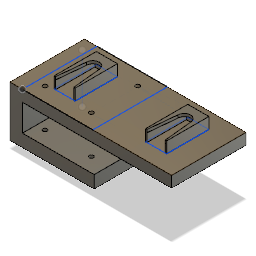
socle stepper 1 (Autodesk Fusion 360 design; units mm, degrees)
Autodesk Fusion 360 part; units mm, degrees
note: some values were not read from the file. Chosen so that the rebuilt part matches the saved one: which face or edge a step refers to. Set by a fixed rule: which sketch regions a step uses.
sketch "Sketch2" plane through (0, 0, 0) normal (0, 1, 0) x (1, 0, 0) in component "junction"
  line L0 (0, 0) -> (100, 0)
  line L1 (100, 0) -> (100, 50)
  line L2 (100, 50) -> (0, 50)
  line L3 (0, 50) -> (0, 0)
  line L4 (100, 50) -> (78.0729, 50)
sketch "Sketch3" plane through (0, 0, 0) normal (1, 0, 0) x (0, 0, -1) in component "junction"
  line L0 (0, 29.5553) -> (50.0119, 29.5553)
  line L1 (50.0119, 29.5553) -> (50.0119, 0)
  line L2 (50.0119, 0) -> (0, 0)
  line L3 (0, 0) -> (0, 29.5553)
sketch "Sketch4" plane through (0, 2.5, -25.0059) normal (1, 0, 0) x (0, 0, -1) in component "junction"
sketch "Sketch5" plane through (0, 0, 0) normal (1, 0, 0) x (0, 1, 0) in component "junction"
  line L0 (30, -50) -> (-5, -50)
extrude "Extrude1" add sketch "Sketch2" along normal blind 10 in component "junction"
extrude "Extrude2" add sketch "Sketch3" along normal blind 5 in component "junction"
extrude "Extrude3" cut 1 faces at (36.6667, 10, -33.3333) along direction (0, -1, 0) blind 5 in component "junction"
extrude "Extrude4" add 1 faces at (36.6667, 5, -33.3333) along direction (0, 1, 0) blind 4 in component "junction"
extrude "Extrude5" add 1 faces at (1.6667, 29.5553, -16.6706) along direction (0, 1, 0) blind 20 in component "junction"
extrude "Extrude6" add 1 faces at (5, 36.0369, -33.3373) along direction (1, 0, 0) blind 4 in component "junction"
extrude "Extrude7" cut 1 faces at (6, 49.5553, -33.3413) along direction (0, -1, 0) blind 10 in component "junction"
extrude "Extrude8" add 1 faces at (6, 39.5553, -33.3413) along direction (0, 1, 0) blind 0.055 in component "junction"
extrude "Extrude9" add 1 faces at (6, 39.6103, -33.3413) along direction (0, 1, 0) blind 0.39 in component "junction"
sketch "Sketch6" plane through (0, 40.0003, 0) normal (0, 1, 0) x (-1, 0, 0) in component "junction"
  line L0 (0, -50.0119) -> (0, 0)
  line L1 (0, 0) -> (-9, 0)
  line L2 (-9, 0) -> (-9, -50.0119)
  line L3 (-9, -50.0119) -> (0, -50.0119)
  line L4 (-9, -50.0119) -> (-115, -50.0119)
  line L5 (-115, -50.0119) -> (-115, 0)
  line L6 (-115, 0) -> (-9, 0)
  line L7 (-9, 0) -> (-9, -50.0119)
  line L8 (-9, 0) -> (-100, 0)
extrude "Extrude10" cut 1 faces at (100, 3, -16.6667) along direction (-1, 0, 0) blind 40 in component "junction"
extrude "Extrude11" add sketch "Sketch6" along normal blind 8 in component "junction"
extrude "Extrude12" add 1 faces at (44.3333, 40.0003, -33.3413) along direction (0, -1, 0) blind 12 in component "junction"
extrude "Extrude13" cut 1 faces at (76.6667, 48.0003, -33.3413) along direction (0, -1, 0) blind 12 in component "junction"
sketch "Sketch7" plane through (0, 0, 0) normal (0, -1, 0) x (1, 0, 0) in component "junction"
  line L0 (60, -50) -> (60, 0)
  line L1 (60, 0) -> (0, 0)
  line L2 (0, 0) -> (0, -50.0119)
  line L3 (0, -50.0119) -> (9, -50.0119)
  line L4 (9, -50.0119) -> (9, -50)
  line L5 (9, -50) -> (60, -50)
  line L6 (50, -5) -> (10, -5)
  line L7 (10, -5) -> (10, -45)
  line L8 (10, -45) -> (50, -45)
  line L9 (50, -45) -> (50, -5)
extrude "Extrude14" cut sketch "Sketch7" against normal blind 5 contours L6 L7 L8 L9 in component "junction"
extrude "Extrude15" cut 1 faces at (50, 3.3333, -31.6667) along direction (1, 0, 0) blind 3 in component "junction"
extrude "Extrude16" cut 1 faces at (38.6667, 1.6667, -45) along direction (0, 0, -1) blind 1.5 in component "junction"
extrude "Extrude17" cut 1 faces at (38.6667, 1.6667, -5) along direction (0, 0, 1) blind 1.5 in component "junction"
extrude "Extrude18" add 1 faces at (3, 21.3335, -50.0119) along direction (0, 0, -1) blind 1.5 in component "junction"
extrude "Extrude19" add 1 faces at (43, 3, -50) along direction (0, 0, -1) blind 1.5 in component "junction"
extrude "Extrude20" add 1 faces at (23, 3, 0) along direction (0, 0, 1) blind 1.5 in component "junction"
sketch "Sketch8" plane through (0, 5, 0) normal (0, -1, 0) x (1, 0, 0) in component "junction"
  line L0 (10, -3.5) -> (10, -46.5)
  line L1 (10, -46.5) -> (53, -46.5)
  line L2 (53, -46.5) -> (53, -3.5)
  line L3 (53, -3.5) -> (10, -3.5)
  line L4 (10, -3.5) -> (53, -46.5)
  line L5 (53, -3.5) -> (10, -46.5)
  circle A0 centre (31.5, -25) radius 11.25
  circle A1 centre (31.5, -25) radius 3
  dimension "d51" = 22.5
  dimension "d52" = 6
  measures "d51" diameter of A0
  measures "d52" diameter of A1
extrude "Extrude21" cut sketch "Sketch8" against normal blind 10 contours L4 L5 A1 | L4 L5 A1 | L4 L5 A1 | L4 L5 A1 in component "junction"
sketch "Sketch9" plane through (0, 5, 0) normal (0, -1, 0) x (1, 0, 0) in component "junction"
  circle A0 centre (31.5, -25) radius 3
  line L0 (10, -3.5) -> (10, -46.5)
  line L1 (10, -46.5) -> (53, -46.5)
  line L2 (53, -46.5) -> (53, -3.5)
  line L3 (53, -3.5) -> (10, -3.5)
  line L4 (10, -3.5) -> (53, -46.5)
  line L5 (53, -3.5) -> (10, -46.5)
  circle A1 centre (31.5, -25) radius 11.25
  dimension "d55" = 22.5
  measures "d55" diameter of A1
extrude "Extrude22" cut sketch "Sketch9" against normal blind 2 contours A0 L4 L5 A1 | A0 L4 L5 A1 | A0 L4 L5 A1 | A0 L4 L5 A1 in component "junction"
sketch "Sketch10" plane through (0, 0, -3.5) normal (0, 0, -1) x (-1, 0, 0) in component "junction"
  line L0 (-53, 0) -> (-10, 0)
  line L1 (-10, 0) -> (-10, 5)
  line L2 (-10, 5) -> (-53, 5)
  line L3 (-53, 5) -> (-53, 0)
sketch "Sketch11" plane through (0, 5, 0) normal (0, -1, 0) x (1, 0, 0) in component "junction"
  circle A0 centre (31.5, -25) radius 11.25
  line L0 (10, -3.5) -> (10, -46.5)
  line L1 (10, -46.5) -> (53, -46.5)
  line L2 (53, -46.5) -> (53, -3.5)
  line L3 (53, -3.5) -> (10, -3.5)
  line L4 (10, -3.5) -> (53, -46.5)
  line L5 (53, -3.5) -> (10, -46.5)
  line L6 (10, -46.5) -> (14, -46.5)
  line L7 (14, -46.5) -> (14, -42.5)
  line L8 (14, -42.5) -> (10, -42.5)
  line L9 (10, -42.5) -> (10, -46.5)
  line L10 (53, -46.5) -> (49, -46.5)
  line L11 (49, -46.5) -> (49, -42.5)
  line L12 (49, -42.5) -> (53, -42.5)
  line L13 (53, -42.5) -> (53, -46.5)
  line L14 (53, -3.5) -> (49, -3.5)
  line L15 (49, -3.5) -> (49, -7.5)
  line L16 (49, -7.5) -> (53, -7.5)
  line L17 (53, -7.5) -> (53, -3.5)
  line L18 (10, -3.5) -> (14, -3.5)
  line L19 (14, -3.5) -> (14, -7.5)
  line L20 (14, -7.5) -> (10, -7.5)
  line L21 (10, -7.5) -> (10, -3.5)
  circle A1 centre (47.9393, -8.5607) radius 1.5
  circle A2 centre (47.9393, -41.4393) radius 1.5
  circle A3 centre (15.0607, -41.4393) radius 1.5
  circle A4 centre (15.0607, -8.5607) radius 1.5
  dimension "d58" = 4
  dimension "d59" = 4
  dimension "d60" = 4
  dimension "d61" = 4
  dimension "d62" = 4
  dimension "d63" = 4
  dimension "d64" = 4
  dimension "d65" = 4
  dimension "d67" = 3
  dimension "d68" = 3
  dimension "d69" = 3
  dimension "d70" = 3
  measures "d67" diameter of A1
  measures "d68" diameter of A2
  measures "d69" diameter of A3
  measures "d70" diameter of A4
extrude "Extrude23" cut sketch "Sketch11" against normal blind 11 contours L5 A3 | L5 A3 in component "junction"
sketch "Sketch12" plane through (0, 5, 0) normal (0, -1, 0) x (1, 0, 0) in component "junction"
  circle A0 centre (15.0607, -41.4393) radius 1.5
  circle A1 centre (31.5, -25) radius 11.25
  line L0 (10, -3.5) -> (10, -46.5)
  line L1 (10, -46.5) -> (53, -46.5)
  line L2 (53, -46.5) -> (53, -3.5)
  line L3 (53, -3.5) -> (10, -3.5)
  line L4 (10, -46.5) -> (53, -3.5)
  line L5 (53, -3.5) -> (49, -3.5)
  line L6 (49, -3.5) -> (49, -7.5)
  line L7 (49, -7.5) -> (53, -7.5)
  line L8 (53, -7.5) -> (53, -3.5)
  circle A2 centre (47.9393, -8.5607) radius 1.5
  dimension "d73" = 4
  dimension "d74" = 4
  dimension "d75" = 3
  measures "d75" diameter of A2
extrude "Extrude24" cut sketch "Sketch12" against normal blind 12 contours L4 A2 | L4 A2 in component "junction"
sketch "Sketch13" plane through (0, 5, 0) normal (0, -1, 0) x (1, 0, 0) in component "junction"
  circle A0 centre (47.9393, -8.5607) radius 1.5
  circle A1 centre (15.0607, -41.4393) radius 1.5
  circle A2 centre (31.5, -25) radius 11.25
  line L0 (10, -3.5) -> (10, -46.5)
  line L1 (10, -46.5) -> (53, -46.5)
  line L2 (53, -46.5) -> (53, -3.5)
  line L3 (53, -3.5) -> (10, -3.5)
  line L4 (10, -3.5) -> (53, -46.5)
  line L5 (10, -3.5) -> (14, -3.5)
  line L6 (14, -3.5) -> (14, -7.5)
  line L7 (14, -7.5) -> (10, -7.5)
  line L8 (10, -7.5) -> (10, -3.5)
  circle A3 centre (15.0607, -8.5607) radius 1.5
  dimension "d78" = 4
  dimension "d79" = 4
  dimension "d80" = 3
  measures "d80" diameter of A3
extrude "Extrude25" cut sketch "Sketch13" against normal blind 15 contours L4 A3 | L4 A3 in component "junction"
sketch "Sketch14" plane through (0, 5, 0) normal (0, -1, 0) x (1, 0, 0) in component "junction"
  circle A0 centre (15.0607, -8.5607) radius 1.5
  circle A1 centre (47.9393, -8.5607) radius 1.5
  circle A2 centre (15.0607, -41.4393) radius 1.5
  circle A3 centre (31.5, -25) radius 11.25
  line L0 (10, -3.5) -> (10, -46.5)
  line L1 (10, -46.5) -> (53, -46.5)
  line L2 (53, -46.5) -> (53, -3.5)
  line L3 (53, -3.5) -> (10, -3.5)
  line L4 (10, -3.5) -> (53, -46.5)
  line L5 (53, -46.5) -> (49, -46.5)
  line L6 (49, -46.5) -> (49, -42.5)
  line L7 (49, -42.5) -> (53, -42.5)
  line L8 (53, -42.5) -> (53, -46.5)
  circle A4 centre (47.9393, -41.4393) radius 1.5
  dimension "d83" = 4
  dimension "d84" = 4
  dimension "d85" = 3
  measures "d85" diameter of A4
extrude "Extrude26" cut sketch "Sketch14" against normal blind 7 contours L4 A4 | L4 A4 in component "junction"
sketch "Sketch15" plane through (0, 5, 0) normal (0, -1, 0) x (1, 0, 0) in component "junction"
  circle A0 centre (47.9393, -41.4393) radius 1.5
  circle A1 centre (15.0607, -8.5607) radius 1.5
  circle A2 centre (47.9393, -8.5607) radius 1.5
  circle A3 centre (15.0607, -41.4393) radius 1.5
  circle A4 centre (31.5, -25) radius 11.25
  line L0 (10, -3.5) -> (10, -46.5)
  line L1 (10, -46.5) -> (53, -46.5)
  line L2 (53, -46.5) -> (53, -3.5)
  line L3 (53, -3.5) -> (10, -3.5)
sketch "Sketch16" plane through (0, 36.0003, 0) normal (0, 1, 0) x (-1, 0, 0) in component "junction"
  line L0 (0, -51.5119) -> (0, 1.5)
  line L1 (0, 1.5) -> (-115, 1.5)
  line L2 (-115, 1.5) -> (-115, -51.5119)
  line L3 (-115, -51.5119) -> (0, -51.5119)
  line L4 (-20, -40) -> (-35, -40)
  line L5 (-35, -40) -> (-35, -10)
  line L6 (-35, -10) -> (-20, -10)
  line L7 (-20, -10) -> (-20, -40)
  line L8 (-100, -40) -> (-85, -40)
  line L9 (-85, -40) -> (-85, -10)
  line L10 (-85, -10) -> (-100, -10)
  line L11 (-100, -10) -> (-100, -40)
  line L12 (-9, 1.5) -> (-59, 1.5)
  line L13 (-59, 1.5) -> (-59, -51.5119)
  line L14 (-59, -51.5119) -> (-9, -51.5119)
  line L15 (-9, -51.5119) -> (-9, 1.5)
  dimension "d88" = 30
  dimension "d89" = 15
  dimension "d90" = 30
  dimension "d91" = 15
  dimension "d114" = 50
  dimension "d115" = 53.0119
  measures "d88" distance of origin
  measures "d90" distance of origin
box "BoxPrimitive2" add length 30 width 15 height 8 placed x (0, 0, 1) y (1, 0, 0) z (0, 1, 0) at (20, 36.0003, -40) in component "junction"
box "BoxPrimitive3" add length 30 width 15 height 8 placed x (0, 0, -1) y (-1, 0, 0) z (0, 1, 0) at (100, 36.0003, -10) in component "junction"
sketch "Sketch18" plane through (0, 36.0003, 0) normal (0, 1, 0) x (-1, 0, 0) in component "junction"
sketch "Sketch19" plane through (0, 44.0003, 0) normal (0, 1, 0) x (-1, 0, 0) in component "junction"
  line L0 (-20, -10) -> (-35, -10)
  line L1 (-35, -10) -> (-35, -40)
  line L2 (-35, -40) -> (-20, -40)
  line L3 (-20, -40) -> (-20, -10)
  line L4 (-20, -40) -> (-35, -10)
  line L5 (-35, -40) -> (-20, -10)
  line L6 (-27.5, -25) -> (-27.5, -40)
  line L7 (-10, -3.5) -> (-10, -46.5)
  line L8 (-13, -30) -> (-43, -30)
  circle A0 centre (-27.5, -30) radius 4.5
  line L9 (-23, -30) -> (-21, -10)
  line L10 (-32, -30) -> (-34, -10)
  dimension "d102" = 9
  measures "d102" diameter of A0
extrude "Extrude27" cut sketch "Sketch19" against normal blind 8 contours L0 L4 L5 L9 L10 | L4 L5 A0 L9 | L4 L8 A0 | L4 L8 A0 | L4 L5 A0 L10 | L4 L6 L8 A0 | L4 L6 L8 A0 | L5 L6 L8 A0 | L5 L8 A0 | L5 L8 A0 | L5 L6 L8 A0 in component "junction"
sketch "Sketch20" plane through (0, 44.0003, 0) normal (0, 1, 0) x (-1, 0, 0) in component "junction"
  line L0 (-100, -40) -> (-85, -40)
  line L1 (-85, -40) -> (-85, -10)
  line L2 (-85, -10) -> (-100, -10)
  line L3 (-100, -10) -> (-100, -40)
  line L4 (-85, -40) -> (-100, -10)
  line L5 (-100, -40) -> (-85, -10)
  line L6 (-70, -30) -> (-108, -30)
  line L7 (-92.5, -25) -> (-92.5, -40)
  circle A0 centre (-92.5, -30) radius 4.5
  line L8 (-88, -30) -> (-86, -10)
  line L9 (-97, -30) -> (-99, -10)
  dimension "d105" = 9
  measures "d105" diameter of A0
extrude "Extrude28" cut sketch "Sketch20" against normal blind 8 contours L5 L6 A0 | L5 L6 L7 A0 | L4 L6 L7 A0 | L5 L6 A0 | L4 L5 A0 L9 | L5 L6 L7 A0 | L4 L6 A0 | L4 L6 L7 A0 | L2 L4 L5 L8 L9 | L5 L7 A0 | L4 L6 A0 | L4 L5 A0 L8 | L4 L7 A0 in component "junction"
extrude "Extrude29" cut 1 faces at (27.5, 44.0003, -25.3339) along direction (0, -1, 0) blind 8 in component "junction"
sketch "Sketch21" plane through (0, 0, -10) normal (0, 0, 1) x (1, 0, 0) in component "junction"
  line L0 (21, 36.0003) -> (21, 44.0003)
  line L1 (21, 44.0003) -> (20, 44.0003)
  line L2 (20, 44.0003) -> (20, 36.0003)
  line L3 (20, 36.0003) -> (21, 36.0003)
  line L4 (21, 42) -> (34, 42)
  line L5 (34, 42) -> (34, 36.0003)
  line L6 (34, 36.0003) -> (21, 36.0003)
  line L7 (21, 36.0003) -> (21, 42)
extrude "Extrude30" cut sketch "Sketch21" against normal blind 28 contours L0 L4 L5 L6 L7 in component "junction"
sketch "Sketch22" plane through (0, 0, -10) normal (0, 0, 1) x (1, 0, 0) in component "junction"
  line L0 (86, 36.0003) -> (86, 44.0003)
  line L1 (86, 44.0003) -> (85, 44.0003)
  line L2 (85, 44.0003) -> (85, 36.0003)
  line L3 (85, 36.0003) -> (86, 36.0003)
  line L4 (86, 42) -> (99, 42)
  line L5 (99, 42) -> (99, 36.0003)
  line L6 (99, 36.0003) -> (86, 36.0003)
  line L7 (86, 36.0003) -> (86, 42)
extrude "Extrude31" cut sketch "Sketch22" against normal blind 28 contours L0 L4 L5 L6 L7 in component "junction"
sketch "Sketch23" plane through (57.5, 36.0003, -25.0059) normal (0, 1, 0) x (-1, 0, 0) in component "junction"
hole "Hole1" at (15.0607, 36.0003, -41.4393) direction (0, -1, 0) diameter 3 depth 11 tip angle 118 in component "junction"
hole "Hole2" at (47.9393, 36.0003, -41.4393) direction (0, -1, 0) diameter 3 depth 11 tip angle 118 in component "junction"
hole "Hole3" at (15.0607, 36.0003, -8.5607) direction (0, -1, 0) diameter 3 depth 11 tip angle 118 in component "junction"
hole "Hole4" at (47.9393, 36.0003, -8.5607) direction (0, -1, 0) diameter 3 depth 11 tip angle 118 in component "junction"
component "junction" placed x (1, 0, 0) y (0, 1, 0) z (0, 0, 1) at (0, 0, 0)
